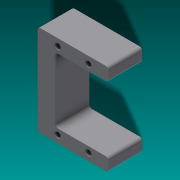
# Autodesk Inventor part: hoefijzer
Saved by Autodesk Inventor 2020.2 (Build 242310000, 310)
## iProperties
Created: 2020-05-19
Part Number: hoefijzer
Material: Generic
Document SubType Name: Modeling
Designer: Svend
Density: 1 g/cm^3
Appearance: Default
Author: Svend
Autodesk Inventor part; units mm, degrees
ref_plane "YZ Plane" through (0, 0, 0) normal (1, 0, 0) x (0, 1, 0)
ref_plane "XZ Plane" through (0, 0, 0) normal (0, 1, 0) x (-1, 0, 0)
ref_plane "XY Plane" through (0, 0, 0) normal (0, 0, 1) x (1, 0, 0)
ref_plane "Work Plane1" through (0, 0, 0) normal (0, 0, 1) x (1, 0, 0)
sketch "Sketch1" plane through (0, 0, 0) normal (0, 0, 1) x (1, 0, 0)
  arc A0 (-2.2638, -13.9278) -> (-4.2638, -11.9278) centre (-4.2638, -13.9278) ccw projected
  line L0 (-42.2638, -11.9278) -> (-4.2638, -11.9278) projected
  arc A1 (-42.2638, -11.9278) -> (-44.2638, -13.9278) centre (-42.2638, -13.9278) ccw projected
  line L1 (-44.2638, -71.9278) -> (-44.2638, -13.9278) projected
  arc A2 (-44.2638, -71.9278) -> (-42.2638, -73.9278) centre (-42.2638, -71.9278) ccw projected
  line L2 (-4.2638, -73.9278) -> (-42.2638, -73.9278) projected
  arc A3 (-4.2638, -73.9278) -> (-2.2638, -71.9278) centre (-4.2638, -71.9278) ccw projected
  line L3 (-2.2638, -13.9278) -> (-2.2638, -71.9278) projected
  circle A4 centre (-23.2638, -42.9278) radius 12.6 projected
  circle A5 centre (-7.2638, -42.9278) radius 2 projected
  circle A6 centre (-23.2638, -58.9278) radius 2 projected
  circle A7 centre (-11.9501, -54.2415) radius 1.5 projected
  circle A8 centre (-34.5775, -54.2415) radius 1.5 projected
  circle A9 centre (-11.9501, -31.6141) radius 1.5 projected
  circle A10 centre (-23.2638, -26.9278) radius 2 projected
  circle A11 centre (-34.5775, -31.6141) radius 1.5 projected
  circle A12 centre (-39.2638, -42.9278) radius 2 projected
  arc A13 (-38.6638, -66.8278) -> (-38.6638, -71.0278) centre (-38.6638, -68.9278) ccw projected
  line L4 (-7.8638, -66.8278) -> (-38.6638, -66.8278) projected
  arc A14 (-7.8638, -71.0278) -> (-7.8638, -66.8278) centre (-7.8638, -68.9278) ccw projected
  line L5 (-38.6638, -71.0278) -> (-7.8638, -71.0278) projected
  arc A15 (-7.8638, -19.0278) -> (-7.8638, -14.8278) centre (-7.8638, -16.9278) ccw projected
  line L6 (-38.6638, -19.0278) -> (-7.8638, -19.0278) projected
  arc A16 (-38.6638, -14.8278) -> (-38.6638, -19.0278) centre (-38.6638, -16.9278) ccw projected
  line L7 (-7.8638, -14.8278) -> (-38.6638, -14.8278) projected
  line L8 (30.6247, -21.3479) -> (-25.1038, -35.8635) projected
  arc A17 (-25.1038, -35.8635) -> (-25.1038, -49.9921) centre (-23.2638, -42.9278) ccw projected
  line L9 (-25.1038, -49.9921) -> (30.6247, -64.5078) projected
  arc A18 (30.6247, -64.5078) -> (30.6247, -21.3479) centre (36.2457, -42.9278) ccw projected
  arc A19 (-24.9022, -36.6377) -> (-24.9022, -49.2179) centre (-23.2638, -42.9278) ccw projected
  line L10 (30.8264, -22.122) -> (-24.9022, -36.6377) projected
  arc A20 (30.8264, -63.7336) -> (30.8264, -22.122) centre (36.2457, -42.9278) ccw projected
  line L11 (-24.9022, -49.2179) -> (30.8264, -63.7336) projected
  line L12 (-44.2638, -20.9278) -> (-2.2638, -20.9278)
  line L13 (-2.2638, -64.9278) -> (-44.2638, -64.9278)
  line L14 (-35.2638, -62.9278) -> (-35.2638, -22.9278)
  line L15 (-47.2638, -13.9278) -> (-47.2638, -71.9278)
  line L16 (-45.2638, -11.9278) -> (-4.2638, -11.9278)
  line L17 (-45.2638, -73.9278) -> (-4.2638, -73.9278)
  arc A21 (-45.2638, -11.9278) -> (-47.2638, -13.9278) centre (-45.2638, -13.9278) ccw
  arc A22 (-47.2638, -71.9278) -> (-45.2638, -73.9278) centre (-45.2638, -71.9278) ccw
  arc A23 (-33.2638, -20.9278) -> (-35.2638, -22.9278) centre (-33.2638, -22.9278) ccw
  arc A24 (-35.2638, -62.9278) -> (-33.2638, -64.9278) centre (-33.2638, -62.9278) ccw
  line L18 (0.7362, -66.9278) -> (0.7362, -71.9278)
  line L19 (0.7362, -13.9278) -> (0.7362, -18.9278)
  line L20 (-2.2638, -20.9278) -> (-1.2638, -20.9278)
  line L21 (-4.2638, -11.9278) -> (-1.2638, -11.9278)
  line L22 (-2.2638, -64.9278) -> (-1.2638, -64.9278)
  line L23 (-4.2638, -73.9278) -> (-1.2638, -73.9278)
  arc A25 (0.7362, -13.9278) -> (-1.2638, -11.9278) centre (-1.2638, -13.9278) ccw
  arc A26 (-1.2638, -20.9278) -> (0.7362, -18.9278) centre (-1.2638, -18.9278) ccw
  arc A27 (0.7362, -66.9278) -> (-1.2638, -64.9278) centre (-1.2638, -66.9278) ccw
  arc A28 (-1.2638, -73.9278) -> (0.7362, -71.9278) centre (-1.2638, -71.9278) ccw
  line L24 (-44.2638, -64.9278) -> (-44.2638, -20.9278)
  point P0 (0, 0)
  point P1 (-35.2638, -20.9278)
  point P2 (-35.2638, -64.9278)
  point P3 (-12.8638, -16.9278)
  point P4 (-33.6638, -16.9278)
  point P5 (-33.6638, -68.9278)
  point P6 (-12.8638, -68.9278)
  point P7 (-35.2638, -55.5753)
  point P8 (-35.2638, -52.9077)
  point P9 (-35.2638, -46.7697)
  point P10 (-35.2638, -39.0859)
  point P11 (-35.2638, -32.9479)
  point P12 (-35.2638, -30.2803)
  point P13 (-47.2638, -11.9278)
  point P14 (-47.2638, -73.9278)
  point P15 (-42.2638, -73.9278)
  point P16 (0.7362, -64.9278)
  point P17 (0.7362, -73.9278)
  point P18 (0.7362, -11.9278)
  point P19 (0.7362, -20.9278)
  dimension "d0" = 9
  dimension "d1" = 9
  dimension "d2" = 9
  dimension "d3" = 5
  dimension "d4" = 5
  dimension "d5" = 5
  dimension "d6" = 5
  dimension "d9" = 3
  dimension "d12" = 3
  dimension "d13" = 3
  constraints: 26 end point, 24 point on line, 16 point on circle, 16 tangent, 12 horizontal alignment, 8 centre point, 8 equal radius, 4 collinear, 3 horizontal, 3 vertical
  measures "d0" distance between parallel lines of L1 L14
  measures "d1" distance between parallel lines of L2 L13
  measures "d2" distance between parallel lines of L0 L12
  measures "d3" distance of point (-33.664, -16.928) A16.centre
  measures "d4" distance of A15.centre point (-12.864, -16.928)
  measures "d5" distance of A14.centre point (-12.864, -68.928)
  measures "d6" distance of A13.centre point (-33.664, -68.928)
  measures "d9" distance between parallel lines of L15 L1
  measures "d12" distance between parallel lines of L18 L3
  measures "d13" distance between parallel lines of L19 L3
extrude "Extrusion1" add sketch "Sketch1" along normal blind 23 contours L3 L12 L1 A1 L0 A0 | A0 L21 A25 L19 A26 L20 L3 | A1 L1 A2 L17 A22 L15 A21 L16 | A23 L14 A11 A4 A8 A24 L13 L1 L12 | L13 L3 A3 L2 A2 L1 | L14 A11 | L22 A27 L18 A28 L23 A3 L3 | L14 A4 | A8 L14 | A12 | L4 A14 L5 A13 | L6 A16 L7 A15 picked at (-35.3642, -31.2378) picked at (-35.3642, -54.6178)
sketch "Sketch2" plane through (0, 0, 23) normal (0, 0, 1) x (1, 0, 0)
  line L0 (-35.2638, -62.9278) -> (-35.2638, -22.9278) projected
  arc A0 (-33.2638, -20.9278) -> (-35.2638, -22.9278) centre (-33.2638, -22.9278) ccw projected
  arc A1 (-1.2638, -20.9278) -> (0.7362, -18.9278) centre (-1.2638, -18.9278) ccw projected
  line L1 (0.7362, -18.9278) -> (0.7362, -13.9278) projected
  arc A2 (0.7362, -13.9278) -> (-1.2638, -11.9278) centre (-1.2638, -13.9278) ccw projected
  line L2 (-1.2638, -11.9278) -> (-45.2638, -11.9278) projected
  arc A3 (-45.2638, -11.9278) -> (-47.2638, -13.9278) centre (-45.2638, -13.9278) ccw projected
  line L3 (-47.2638, -13.9278) -> (-47.2638, -71.9278) projected
  arc A4 (-47.2638, -71.9278) -> (-45.2638, -73.9278) centre (-45.2638, -71.9278) ccw projected
  line L4 (-45.2638, -73.9278) -> (-1.2638, -73.9278) projected
  arc A5 (-1.2638, -73.9278) -> (0.7362, -71.9278) centre (-1.2638, -71.9278) ccw projected
  line L5 (0.7362, -71.9278) -> (0.7362, -66.9278) projected
  arc A6 (0.7362, -66.9278) -> (-1.2638, -64.9278) centre (-1.2638, -66.9278) ccw projected
  line L6 (-1.2638, -64.9278) -> (-33.2638, -64.9278) projected
  arc A7 (-35.2638, -62.9278) -> (-33.2638, -64.9278) centre (-33.2638, -62.9278) ccw projected
  line L7 (-33.2638, -20.9278) -> (-1.2638, -20.9278) projected
  point P0 (0, 0)
  point P1 (-12.8638, -16.9278)
  point P2 (-33.6638, -16.9278)
  point P3 (-33.6638, -68.9278)
  point P4 (-12.8638, -68.9278)
hole "Hole1" at (-12.8638, -16.9278, 23) at (-33.6638, -16.9278, 23) at (-33.6638, -68.9278, 23) at (-12.8638, -68.9278, 23) direction (0, 0, -1) diameter 3.242 end through all thread size "M4x0.7" class "6H" standard "ISO Metric profile"
chamfer "Chamfer1" distance 0.5 angle 45 8 edges at (-12.8638, -15.3068, 23) (-33.6638, -15.3068, 23) (-33.6638, -67.3068, 23) (-12.8638, -67.3068, 23) (-12.8638, -67.3068, 0) (-33.6638, -67.3068, 0) (-33.6638, -15.3068, 0) (-12.8638, -15.3068, 0)
equation "\"d1\" = d2"
equation "\"d2\" = d0"
equation "\"d4\" = d3"
equation "\"d5\" = d4"
equation "\"d6\" = d5"
equation "\"d12\" = d9"
equation "\"d13\" = d12"
body "Solid1"
